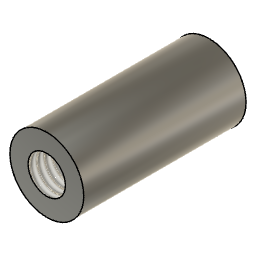
Spacer v2 (Autodesk Fusion 360 design; units mm, degrees)
Autodesk Fusion 360 part; units mm, degrees
sketch "Sketch1" plane through (0, 0, 0) normal (0, 1, 0) x (1, 0, 0)
  circle A0 centre (0, 0) radius 2.5
  dimension "d1" = 5
  constraint coincident A0.centre origin
  measures "d1" diameter of A0
extrude "Extrude2" add sketch "Sketch1" along normal blind 11
hole "Hole2" at (-0.0071, 0, 0.0022) direction (0, 1, 0) diameter 2.529 end through all
thread "Thread2" "ISO Metric profile 3.0 M3x0.5 6H" thread offset 0 thread depth 7.4
